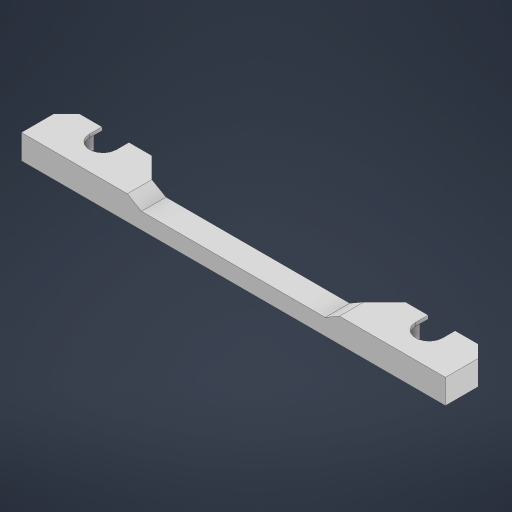
# Autodesk Inventor part: miniboard nutt holder
Saved by Autodesk Inventor 2024 (Build 280153000, 153)
## iProperties
Created: 2024-03-17
Part Number: miniboard nutt holder
Material: Všeobecné
Document SubType Name: Modeling
Designer: Simak
Density: 1 g/cm^3
Appearance: Výchozí
Author: Simak
Autodesk Inventor part; units mm, degrees
ref_plane "YZ Plane" through (0, 0, 0) normal (1, 0, 0) x (0, 1, 0)
ref_plane "XZ Plane" through (0, 0, 0) normal (0, 1, 0) x (-1, 0, 0)
ref_plane "XY Plane" through (0, 0, 0) normal (0, 0, 1) x (1, 0, 0)
sketch "Náčrt1" plane through (0, 0, 0) normal (0, 1, 0) x (-1, 0, 0)
  line L0 (14, -2) -> (10.9112, 1.0888)
  line L1 (10.9112, 1.0888) -> (-10.9112, 1.0888)
  line L2 (-10.9112, 1.0888) -> (-14, -2)
  line L3 (-14, -2) -> (-26, -2)
  line L4 (-26, -2) -> (-26, 2)
  line L5 (-26, 2) -> (26, 2)
  line L6 (26, 2) -> (26, -2)
  line L7 (26, -2) -> (14, -2)
  line L8 (20, 1.0888) -> (22.675, -0.4556)
  line L9 (22.675, -0.4556) -> (22.675, -3.5444)
  line L10 (22.675, -3.5444) -> (20, -5.0888)
  line L11 (20, -5.0888) -> (17.325, -3.5444)
  line L12 (17.325, -3.5444) -> (17.325, -0.4556)
  line L13 (17.325, -0.4556) -> (20, 1.0888)
  line L14 (-20, 1.0888) -> (-17.325, -0.4556)
  line L15 (-17.325, -0.4556) -> (-17.325, -3.5444)
  line L16 (-17.325, -3.5444) -> (-20, -5.0888)
  line L17 (-20, -5.0888) -> (-22.675, -3.5444)
  line L18 (-22.675, -3.5444) -> (-22.675, -0.4556)
  line L19 (-22.675, -0.4556) -> (-20, 1.0888)
  line L20 (26, 2) -> (0, 0) construction
  line L21 (0, 0) -> (-26, 2) construction
  line L22 (26, -2) -> (0, 0) construction
  line L23 (-17.325, -3.5444) -> (-15.5444, -3.5444)
  line L24 (-15.5444, -3.5444) -> (-14, -2)
  line L25 (17.325, -3.5444) -> (15.5444, -3.5444)
  line L26 (15.5444, -3.5444) -> (14, -2)
  line L27 (-22.675, -3.5444) -> (-24.4556, -3.5444)
  line L28 (-24.4556, -3.5444) -> (-26, -2)
  line L29 (22.675, -3.5444) -> (24.4556, -3.5444)
  line L30 (24.4556, -3.5444) -> (26, -2)
  line L31 (-13, -1) -> (13, -1)
  point P0 (20, -2)
  point P1 (-20, -2)
  dimension "d0" = 5.35
  dimension "d1" = 40
  dimension "d4" = 4
  dimension "d6" = 45
  dimension "d7" = 1
  dimension "d8" = 52
  constraints: 64 end point, 8 equal length, 8 horizontal, 4 vertical, 3 point on line, 2 collinear, 2 midpoint, 1 parallel, 26 other
  measures "d0" distance between parallel lines of L12 L9
  measures "d1" distance of point (20, -2) point (-20, -2)
  measures "d4" distance between parallel lines of L5 L3
  measures "d6" angle of L7 L30
  measures "d7" distance between parallel lines of L31 L3
  measures "d8" distance between parallel lines of L4 L6
extrude "Vysunutí1" add sketch "Náčrt1" along normal blind 3 contours L0 L1 L2 L3 L15 L14 L19 L18 L4 L5 L6 L7 L9 L8 L13 L12 | L7 L12 L25 L26 | L31 L2 L1 L0 | L7 L30 L29 L9 | L24 L23 L15 L3 | L18 L27 L28 L3
sketch "Náčrt2" plane through (0, 3, 0) normal (0, 1, 0) x (1, 0, 0)
  line L0 (-13, 1) -> (-15.5444, 3.5444) projected
  line L1 (-15.5444, 3.5444) -> (-17.325, 3.5444) projected
  line L2 (-17.325, 3.5444) -> (-17.325, 0.4556) projected
  line L3 (-17.325, 0.4556) -> (-20, -1.0888) projected
  line L4 (-20, -1.0888) -> (-22.675, 0.4556) projected
  line L5 (-22.675, 0.4556) -> (-22.675, 3.5444) projected
  line L6 (-22.675, 3.5444) -> (-24.4556, 3.5444) projected
  line L7 (-24.4556, 3.5444) -> (-26, 2) projected
  line L8 (-26, 2) -> (-26, -2) projected
  line L9 (-26, -2) -> (26, -2) projected
  line L10 (26, -2) -> (26, 2) projected
  line L11 (26, 2) -> (24.4556, 3.5444) projected
  line L12 (24.4556, 3.5444) -> (22.675, 3.5444) projected
  line L13 (22.675, 3.5444) -> (22.675, 0.4556) projected
  line L14 (22.675, 0.4556) -> (20, -1.0888) projected
  line L15 (20, -1.0888) -> (17.325, 0.4556) projected
  line L16 (17.325, 0.4556) -> (17.325, 3.5444) projected
  line L17 (17.325, 3.5444) -> (15.5444, 3.5444) projected
  line L18 (15.5444, 3.5444) -> (13, 1) projected
  line L19 (13, 1) -> (-13, 1) projected
  circle A0 centre (-20, 2) radius 1.65
  circle A1 centre (20, 2) radius 1.65
  line L20 (-22.675, 0.4556) -> (-20, 2) construction
  line L21 (-20, 2) -> (-17.325, 0.4556) construction
  line L22 (-20, 2) -> (-20, -1.0888) construction
  line L23 (20, 2) -> (22.675, 0.4556) construction
  line L24 (20, -1.0888) -> (20, 2) construction
  line L25 (17.325, 0.4556) -> (20, 2) construction
  line L26 (-22.675, 3.5444) -> (-17.325, 3.5444)
  line L27 (22.675, 3.5444) -> (17.325, 3.5444)
  line L28 (18.35, 2) -> (18.35, 3.5444)
  line L29 (21.65, 2) -> (21.65, 3.5444)
  line L30 (-18.35, 2) -> (-18.35, 3.5444)
  line L31 (-21.65, 2) -> (-21.65, 3.5444)
  point P0 (0, 0)
  dimension "d11" = 3.3
  constraints: 24 end point, 7 equal length, 4 perpendicular, 4 point on circle, 4 point on line, 4 tangent, 2 centre point, 1 equal radius, 1 horizontal, 1 vertical
  measures "d11" diameter of A0
extrude "Vysunutí2" add sketch "Náčrt2" against normal blind 0.4 contours L2 L3 L4 L5 L26 L31 A0 L30 | L27 L28 A1 L29 L13 L14 L15 L16
sketch "Náčrt3" plane through (13, 0, -1) normal (0, 0, -1) x (-1, 0, 0)
  line L0 (0, 0) -> (26, 0) projected
  line L1 (26, 0) -> (26, 3) projected
  line L2 (0, 3) -> (26, 3) projected
  line L3 (0, 0) -> (0, 3) projected
  line L4 (0, 3) -> (1.7321, 2)
  line L5 (1.7321, 2) -> (24.2679, 2)
  line L6 (24.2679, 2) -> (26, 3)
  point P0 (13, 0)
  dimension "d14" = 2
  dimension "d16" = 60
  constraints: 6 end point, 1 equal length, 1 horizontal
  measures "d14" distance between parallel lines of L0 L5
  measures "d16" angle of L3 L4
extrude "Vysunutí3" cut sketch "Náčrt3" against normal through all contours L2 L6 L5 L4
